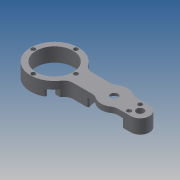
# Autodesk Inventor part: SCREW BOTTOM ARM
Saved by Autodesk Inventor 2013 (Build 170138000, 138)
## iProperties
Created: 2017-04-04
Part Number: SCREW BOTTOM ARM
Material: Generic
Document SubType Name: Modeling
Designer: employee
Density: 1 g/cm^3
Author: employee
Autodesk Inventor part; units mm, degrees
ref_plane "YZ Plane" through (0, 0, 0) normal (1, 0, 0) x (0, 1, 0)
ref_plane "XZ Plane" through (0, 0, 0) normal (0, 1, 0) x (-1, 0, 0)
ref_plane "XY Plane" through (0, 0, 0) normal (0, 0, 1) x (1, 0, 0)
sketch "Sketch1" plane through (0, 0, 0) normal (0, 0, 1) x (1, 0, 0)
  line L0 (0, 12.5) -> (115.5, 12.5)
  arc A0 (115.5, -12.5) -> (115.5, 12.5) centre (115.5, 0) ccw
  line L1 (115.5, -12.5) -> (0, -12.5)
  arc A1 (0, 12.5) -> (0, -12.5) centre (0, 0) ccw
  circle A2 centre (115.5, 0) radius 6
  dimension "d0" = 115.5
  dimension "d2" = 12.5
  dimension "d3" = 12
  constraints: 4 end point, 4 point on circle, 4 tangent, 3 centre point, 2 coincident, 1 horizontal, 1 parallel
  measures "d0" distance of L1.start L1.end
  measures "d2" radius of A1
  measures "d3" diameter of A2
extrude "Extrusion1" add sketch "Sketch1" along normal mid plane 38
sketch "Sketch2" plane through (0, 0, 19) normal (0, 0, 1) x (1, 0, 0)
  circle A0 centre (115.5, 0) radius 6 projected
  circle A1 centre (80.5, 0) radius 22.2817 construction
  circle A2 centre (80.5, 0) radius 5
  dimension "d6" = 44.5634
  dimension "d8" = 35
  dimension "d9" = 10
  constraints: 2 centre point, 1 coincident, 1 horizontal alignment
  measures "d6" diameter of A1
  measures "d8" distance of A1.centre A0.centre
  measures "d9" diameter of A2
extrude "Extrusion2" cut sketch "Sketch2" against normal through all contours A2
sketch "Sketch3" plane through (0, 0, 0) normal (0, 0, 1) x (1, 0, 0)
  circle A0 centre (80.5, 0) radius 5 projected
  circle A1 centre (115.5, 0) radius 6 projected
  arc A2 (115.5, -12.5) -> (115.5, 12.5) centre (115.5, 0) ccw projected
  line L0 (115.5, -12.5) -> (0, -12.5) projected
  arc A3 (0, 12.5) -> (0, -12.5) centre (0, 0) ccw projected
  line L1 (0, 12.5) -> (115.5, 12.5) projected
  circle A4 centre (80.5, 0) radius 25
  dimension "d12" = 50
  constraints: 1 centre point, 1 coincident
  measures "d12" diameter of A4
extrude "Extrusion3" cut sketch "Sketch3" along normal mid plane 23 contours A4 L0 | L0 A4 L1 | L1 A4
sketch "Sketch4" plane through (0, 0, -11.5) normal (0, 0, 1) x (1, 0, 0)
  circle A0 centre (80.5, 0) radius 5 projected
  circle A1 centre (80.5, 0) radius 10.5
  point P0 (0, 0)
  dimension "d16" = 21
  constraints: 1 centre point, 1 coincident
  measures "d16" diameter of A1
extrude "Extrusion4" cut sketch "Sketch4" against normal blind 4
sketch "Sketch5" plane through (0, 0, -11.5) normal (0, 0, 1) x (1, 0, 0)
  circle A0 centre (80.5, 0) radius 10.5 projected
  arc A1 (58.8494, 12.5) -> (58.8494, -12.5) centre (80.5, 0) ccw projected
  circle A2 centre (80.5, 0) radius 18
  point P0 (0, 0)
  dimension "d22" = 7.5
  constraints: 1 centre point, 1 coincident
  measures "d22" radial gap between concentric circles of A2 A0
extrude "Extrusion5" add sketch "Sketch5" against normal up to surface (7.5 mm away)
mirror "Mirror1" about plane through (0, 0, 0) normal (0, 0, 1) of "Extrusion4", "Extrusion5"
sketch "Sketch6" plane through (0, 0, -19) normal (0, 0, -1) x (-1, 0, 0)
  arc A0 (-115.5, 12.5) -> (-115.5, -12.5) centre (-115.5, 0) ccw projected
  line L0 (-67.5482, 12.5) -> (0, 12.5) projected
  circle A1 centre (-80.5, 0) radius 10.5 projected
  line L1 (-58.8494, -12.5) -> (-67.5482, -12.5) projected
  arc A2 (-58.8494, -12.5) -> (-58.8494, 12.5) centre (-80.5, 0) ccw projected
  line L2 (-67.5482, 12.5) -> (-58.8494, 12.5) projected
  arc A3 (-67.5482, 12.5) -> (-93.4518, 12.5) centre (-80.5, 0) ccw projected
  line L3 (-102.1506, 12.5) -> (-93.4518, 12.5) projected
  arc A4 (-102.1506, 12.5) -> (-102.1506, -12.5) centre (-80.5, 0) ccw projected
  line L4 (-93.4518, -12.5) -> (-102.1506, -12.5) projected
  arc A5 (-93.4518, -12.5) -> (-67.5482, -12.5) centre (-80.5, 0) ccw projected
  circle A6 centre (-108, -7.5) radius 1.5
  circle A7 centre (-108, 7.5) radius 1.5
  dimension "d25" = 3
  dimension "d27" = 7.5
  dimension "d28" = 7.5
  dimension "d29" = 7.5
  dimension "d30" = 7.5
  constraints: 2 centre point, 1 equal radius
  measures "d25" diameter of A7
  measures "d27" horizontal distance of A7.centre A0.centre
  measures "d28" horizontal distance of A7.centre A0.centre
  measures "d29" horizontal distance of A6.centre A0.centre
  measures "d30" horizontal distance of A0.centre A6.centre
extrude "Extrusion6" cut sketch "Sketch6" against normal through all contours A6 | A7
sketch "Sketch7" plane through (0, 0, 19) normal (0, 0, 1) x (1, 0, 0)
  circle A0 centre (108, 7.5) radius 1.5 projected
  circle A1 centre (108, -7.5) radius 1.5 projected
  circle A2 centre (80.5, 0) radius 5 projected
  line L0 (108.8355, 4.4365) -> (105.7647, 5.2447)
  line L1 (105.7647, 5.2447) -> (104.9291, 8.3082)
  line L2 (104.9291, 8.3082) -> (107.1645, 10.5635)
  line L3 (107.1645, 10.5635) -> (110.2353, 9.7553)
  line L4 (110.2353, 9.7553) -> (111.0709, 6.6918)
  line L5 (111.0709, 6.6918) -> (108.8355, 4.4365)
  line L6 (105.7647, -5.2447) -> (108.8355, -4.4365)
  line L7 (108.8355, -4.4365) -> (111.0709, -6.6918)
  line L8 (111.0709, -6.6918) -> (110.2353, -9.7553)
  line L9 (110.2353, -9.7553) -> (107.1645, -10.5635)
  line L10 (107.1645, -10.5635) -> (104.9291, -8.3082)
  line L11 (104.9291, -8.3082) -> (105.7647, -5.2447)
  line L12 (80.5, 0) -> (108, -7.5) construction
  dimension "d92" = 5.5
  constraints: 26 end point, 2 coincident, 1 equal length, 1 perpendicular, 1 vertical alignment, 26 other
  measures "d92" distance between parallel lines of L5 L2
extrude "Extrusion7" cut sketch "Sketch7" against normal blind 4 contours L0 L1 L2 L3 L4 L5 | L6 L7 L8 L9 L10 L11
sketch "Sketch9" plane through (0, 0, -19) normal (0, 0, -1) x (-1, 0, 0)
  circle A0 centre (-115.5, 0) radius 6 projected
  circle A1 centre (-115.5, 0) radius 5
  dimension "d43" = 1
  constraints: 1 centre point
  measures "d43" radial gap between concentric circles of A1 A0
extrude "Extrusion9" add sketch "Sketch9" against normal blind 1.5
sketch "Sketch10" plane through (0, 0, 19) normal (0, 0, 1) x (1, 0, 0)
  circle A0 centre (115.5, 0) radius 6 projected
  circle A1 centre (115.5, 0) radius 5 projected
extrude "Extrusion10" add sketch "Sketch10" against normal blind 1.5
sketch "Sketch11" plane through (0, 0, 19) normal (0, 0, 1) x (1, 0, 0)
  arc A0 (0, 12.5) -> (0, -12.5) centre (0, 0) ccw projected
  circle A1 centre (0, 0) radius 25
  circle A2 centre (0, 0) radius 32.5
  dimension "d50" = 65
  dimension "d51" = 7.5
  constraints: 2 centre point, 2 coincident
  measures "d50" diameter of A2
  measures "d51" radial gap between concentric circles of A2 A1
extrude "Extrusion11" add sketch "Sketch11" against normal up to surface (38 mm away)
sketch "Sketch12" plane through (0, 0, -19) normal (0, 0, -1) x (-1, 0, 0)
  arc A0 (-21.6506, -12.5) -> (-21.6506, 12.5) centre (0, 0) ccw projected
  line L0 (-21.6506, -12.5) -> (0, -12.5) projected
  arc A1 (0, -12.5) -> (0, 12.5) centre (0, 0) ccw projected
  line L1 (0, 12.5) -> (-21.6506, 12.5) projected
  circle A2 centre (0, 0) radius 25
  constraints: 1 coincident, 3 other
extrude "Extrusion12" cut sketch "Sketch12" against normal through all contours A2 L1 A1 L0
sketch "Sketch13" plane through (0, 0, 19) normal (0, 0, 1) x (1, 0, 0)
  circle A0 centre (0, 0) radius 25 projected
  circle A1 centre (0, 0) radius 25
  constraints: 1 centre point, 1 coincident, 1 concentric
extrude "Extrusion13" add sketch "Sketch13" against normal blind 11.4
sketch "Sketch14" plane through (0, 0, -19) normal (0, 0, -1) x (-1, 0, 0)
  circle A0 centre (0, 0) radius 25 projected
  line L0 (-30, 12.5) -> (-67.5482, 12.5) projected
  arc A1 (-67.5482, 12.5) -> (-93.4518, 12.5) centre (-80.5, 0) ccw projected
  line L1 (-93.4518, 12.5) -> (-115.5, 12.5) projected
  arc A2 (-115.5, 12.5) -> (-115.5, -12.5) centre (-115.5, 0) ccw projected
  line L2 (-115.5, -12.5) -> (-93.4518, -12.5) projected
  arc A3 (-93.4518, -12.5) -> (-67.5482, -12.5) centre (-80.5, 0) ccw projected
  line L3 (-67.5482, -12.5) -> (-30, -12.5) projected
  arc A4 (-30, -12.5) -> (-30, 12.5) centre (0, 0) ccw projected
  circle A5 centre (-80.5, 0) radius 5 projected
  circle A6 centre (-108, 7.5) radius 1.5 projected
  circle A7 centre (-108, -7.5) radius 1.5 projected
  circle A8 centre (-115.5, 0) radius 5 projected
extrude "Extrusion14" cut sketch "Sketch14" against normal up to surface (19 mm away)
sketch "Sketch17" plane through (0, 0, 7.6) normal (0, 0, -1) x (-1, 0, 0)
  circle A0 centre (0, 0) radius 11 projected
  circle A1 centre (-80.5, 0) radius 5 projected
  circle A2 centre (-80.5, 0) radius 22.0277
  line L0 (0, 19.0554) -> (-80.5, 19.0554)
  line L1 (-80.5, 19.0554) -> (-80.5, 25)
  line L2 (-80.5, 25) -> (0, 25)
  line L3 (0, 25) -> (0, 19.0554)
  line L4 (-80.5, -19.0554) -> (0, -19.0554)
  line L5 (0, -19.0554) -> (0, -25)
  line L6 (0, -25) -> (-80.5, -25)
  line L7 (-80.5, -25) -> (-80.5, -19.0554)
  circle A3 centre (0, 0) radius 25 projected
  point P0 (-80.5, 22.0277)
  point P1 (-80.5, -22.0277)
  dimension "d68" = 44.0554
  constraints: 16 end point, 4 parallel, 4 vertical alignment, 2 horizontal, 2 midpoint, 2 perpendicular, 2 point on circle, 1 centre point, 1 coincident, 1 collinear, 1 tangent
  measures "d68" diameter of A2
extrude "Extrusion17" cut sketch "Sketch17" along normal through all contours L0 L1 A2 | A2 L1 L2 A3 L0 | L4 A3 L6 L7 A2 | A2 L7 L4 | A3 L3 L0 | L4 L5 A3
sketch "Sketch18" plane through (0, 0, 7.6) normal (0, 0, -1) x (-1, 0, 0)
  arc A0 (-16.183, 19.0554) -> (-16.183, -19.0554) centre (0, 0) ccw projected
  circle A1 centre (0, 22.5) radius 1.75
  circle A2 centre (0, 28.75) radius 1.75
  dimension "d73" = 28.75
  dimension "d74" = 22.5
  dimension "d75" = 3.5
  constraints: 2 centre point, 2 vertical alignment, 1 equal radius
  measures "d73" distance of A2.centre A0.centre
  measures "d74" distance of A1.centre A0.centre
  measures "d75" diameter of A1
extrude "Extrusion18" cut sketch "Sketch18" along normal through all both and the other way through all
pattern_circular "Circular Pattern2" count 4 over 360 about axis through (0, 0, 19) along (0, 0, -1) of "Extrusion18"
sketch "Sketch20" plane through (0, 0, 19) normal (0, 0, 1) x (1, 0, 0)
  circle A0 centre (-28.75, 0) radius 1.75 projected
  circle A1 centre (0, -28.75) radius 1.75 projected
  circle A2 centre (28.75, 0) radius 1.75 projected
  circle A3 centre (0, 28.75) radius 1.75 projected
  line L0 (-3.1754, 28.75) -> (-1.5877, 31.5)
  line L1 (-1.5877, 31.5) -> (1.5877, 31.5)
  line L2 (1.5877, 31.5) -> (3.1754, 28.75)
  line L3 (3.1754, 28.75) -> (1.5877, 26)
  line L4 (1.5877, 26) -> (-1.5877, 26)
  line L5 (-1.5877, 26) -> (-3.1754, 28.75)
  dimension "d95" = 5.5
  constraints: 12 end point, 1 coincident, 1 horizontal, 13 other
  measures "d95" distance between parallel lines of L4 L1
extrude "Extrusion20" cut sketch "Sketch20" against normal blind 4 contours L0 L1 L2 L3 L4 L5
fillet "Fillet1" radius 2 10 edges at (16.183, 19.0554, 3.8) (20.7666, 25, 3.8) (26.3276, 19.0554, 3.8) (16.183, -19.0554, 3.8) (26.3276, -19.0554, 3.8) (20.7666, -25, 3.8) (58.8494, -12.5, 5.75) (58.8494, 12.5, 5.75) (102.1506, 12.5, 5.75) (102.1506, -12.5, 5.75)
fillet "Fillet2" radius 12.5 6 edges at (93.4518, 12.5, 15.25) (67.5482, 12.5, 15.25) (67.5482, -12.5, 15.25) (93.4518, -12.5, 15.25) (30, -12.5, 9.5) (30, 12.5, 9.5)
sketch "Sketch21" plane through (0, 0, 7.6) normal (0, 0, -1) x (-1, 0, 0)
  circle A0 centre (22.5, 0) radius 1.75 projected
  circle A1 centre (0, -22.5) radius 1.75 projected
  circle A2 centre (-22.5, 0) radius 1.75 projected
  circle A3 centre (0, 22.5) radius 1.75 projected
  arc A4 (-19.3807, 15.7921) -> (-19.3807, -15.7921) centre (0, 0) ccw projected
  circle A5 centre (0, 0) radius 25
  constraints: 1 coincident, 3 other
extrude "Extrusion21" cut sketch "Sketch21" against normal through all
pattern_circular "Circular Pattern3" count 4 over 360 about axis through (0, 0, 19) along (0, 0, -1) of "Extrusion20"
sketch "Sketch22" plane through (80.5, 0, 15.5) normal (0, 0, -1) x (-1, 0, 0)
  circle A0 centre (0, 0) radius 5 projected
  circle A1 centre (0, 0) radius 10.5 projected
  circle A2 centre (0, 0) radius 9.5
  point P0 (80.5, 0)
  dimension "d99" = 1
  constraints: 1 centre point, 1 coincident
  measures "d99" radial gap between concentric circles of A1 A2
extrude "Extrusion22" cut sketch "Sketch22" against normal blind 1 contours A2
body "Solid1"
